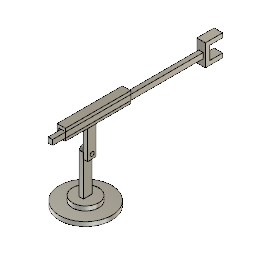
Modelling and Simulation of a Polar Robot (RRP) (Autodesk Fusion 360 design; units mm, degrees)
Autodesk Fusion 360 part; units mm, degrees
sketch "Sketch1" plane through (0, 0, 0) normal (0, 0, 1) x (1, 0, 0)
  circle A0 centre (0, 0) radius 60
  dimension "d1" = 120
  constraint coincident A0.centre origin
  measures "d1" diameter of A0
extrude "Extrude1" add sketch "Sketch1" along normal blind 10 makes body 1 in component "Component"
sketch "Sketch2" plane through (0, 0, 10) normal (0, 0, 1) x (-1, 0, 0)
  circle A0 centre (0, 0) radius 60
  circle A1 centre (0, 0) radius 30
  dimension "d4" = 60
  constraint coincident A0.centre A1.centre
  measures "d4" diameter of A1
extrude "Extrude1'" add sketch "Sketch2" along normal blind 10 separate body contours A1 makes body 2 in component "Component'"
sketch "Sketch3" plane through (0, 0, 20) normal (0, 0, 1) x (-1, 0, 0)
  circle A0 centre (0, 0) radius 30
  line L0 (-5, 10) -> (5, 10)
  line L1 (5, 10) -> (5, -10)
  line L2 (5, -10) -> (-5, -10)
  line L3 (-5, -10) -> (-5, 10)
  line L4 (-5, 10) -> (5, -10) construction
  line L5 (5, 10) -> (-5, -10) construction
  dimension "d7" = 20
  dimension "d8" = 10
  dimension "d9" = 10
  dimension "d10" = 20
  constraint horizontal L0
  constraint perpendicular L0 L1
  constraint parallel L0 L2
  constraint parallel L1 L3
  constraint coincident L4 A0.centre
  constraint coincident L5 A0.centre
  constraint coincident A0.centre origin
  measures "d7" distance of L0.end L1.end
  measures "d8" distance of L1.end L2.end
  measures "d9" distance of L1.end L2.end
  measures "d10" distance of L0.end L1.end
extrude "Extrude2" add sketch "Sketch3" along normal blind 100 contours L0 L1 L2 L3 bodies 2 in component "Component'"
sketch "Sketch4" plane through (-5, 0, 0) normal (-1, 0, 0) x (0, -1, 0)
  line L0 (-10, 20) -> (10, 20)
  line L1 (10, 20) -> (10, 120)
  line L2 (10, 120) -> (-10, 120)
  line L3 (-10, 120) -> (-10, 20)
  arc A0 (10, 106.2063) -> (-10, 105.8869) centre (-0.0542, 109.439) ccw
  line L4 (-10, 105.8869) -> (-10, 120)
  line L5 (10, 120) -> (10, 106.2063)
  constraint coincident L1 A0.start
  constraint coincident L3 A0.end
  constraint coincident L2.end L3.start
  constraint coincident L1.end L2.start
extrude "Extrude3" cut sketch "Sketch4" against normal blind 70 contours L2 L3 A0 L4 | L1 L2 A0 L5 bodies 2 in component "Component'"
sketch "Sketch5" plane through (5, 0, 0) normal (1, 0, 0) x (0, 1, 0)
  arc A0 (10, 112.9912) -> (0.1084, 120) centre (0.0542, 109.439) ccw
  line L0 (0.1084, 120) -> (0, 120)
  arc A1 (0, 120) -> (-10, 112.6717) centre (0.0542, 109.439) ccw
  line L1 (-10, 112.6717) -> (-10, 20)
  line L2 (-10, 20) -> (10, 20)
  line L3 (10, 20) -> (10, 112.9912)
  circle A2 centre (0.0542, 109.439) radius 4.5
  dimension "d15" = 9
  constraint concentric A0 A2
  measures "d15" diameter of A2
extrude "Extrude4" add sketch "Sketch5" along normal blind 10 contours A2 bodies 2 in component "Component'"
sketch "Sketch6" plane through (15, 0, 0) normal (1, 0, 0) x (0, 1, 0)
  circle A0 centre (0.0542, 109.439) radius 4.5
  line L0 (-10, 120) -> (60, 120)
  line L1 (60, 120) -> (60, 100)
  line L2 (60, 100) -> (-10, 100)
  line L3 (-10, 100) -> (-10, 120)
  constraint horizontal L0
  constraint vertical L1
  constraint horizontal L2
  constraint vertical L3
extrude "Extrude1''" add sketch "Sketch6" against normal blind 10 separate body makes body 3 in component "Component''"
sketch "Sketch7" plane through (0, 9.4932, 0) normal (0, 1, 0) x (-1, 0, 0)
  line L0 (-15, 169.3849) -> (-15, 99.3849)
  line L1 (-15, 99.3849) -> (-5, 99.3849)
  line L2 (-5, 99.3849) -> (-5, 169.3849)
  line L3 (-5, 169.3849) -> (-15, 169.3849)
  line L4 (-19.341, 169.3448) -> (0.1035, 169.3448)
  line L5 (0.1035, 169.3448) -> (0.1035, 195.3844)
  line L6 (0.1035, 195.3844) -> (-19.341, 195.3844)
  line L7 (-19.341, 195.3844) -> (-19.341, 169.3448)
  line L8 (-19.341, 169.3448) -> (0.1035, 195.3844) construction
  line L9 (0.1035, 169.3448) -> (-19.341, 195.3844) construction
  point P0 (-9.6187, 182.3646)
  constraint horizontal L4
  constraint perpendicular L4 L5
  constraint parallel L4 L6
  constraint parallel L5 L7
  constraint coincident L8 P0
  constraint coincident L9 P0
extrude "Extrude2'" add sketch "Sketch7" along normal mid plane 150 contours L0 L2 L3 L4 L5 L6 L7 sketch seen with x (1, 0, 0) y (0, 0, -1) z (0, 1, 0) at (0, -109.3849, 109.4932) bodies 3 in component "Component''"
sketch "Sketch8" plane through (0, 84.4932, 0) normal (0, 1, 0) x (-1, 0, 0)
  line L0 (-5, 169.3448) -> (0.1035, 169.3448)
  line L1 (0.1035, 169.3448) -> (0.1035, 195.3844)
  line L2 (0.1035, 195.3844) -> (-19.341, 195.3844)
  line L3 (-19.341, 195.3844) -> (-19.341, 169.3448)
  line L4 (-19.341, 169.3448) -> (-15, 169.3448)
  line L5 (-15, 169.3448) -> (-15, 169.3849)
  line L6 (-15, 169.3849) -> (-5, 169.3849)
  line L7 (-5, 169.3849) -> (-5, 169.3448)
  line L8 (-4.1596, 176.2347) -> (-14.668, 176.2347)
  line L9 (-14.668, 176.2347) -> (-14.668, 188.4945)
  line L10 (-14.668, 188.4945) -> (-4.1596, 188.4945)
  line L11 (-4.1596, 188.4945) -> (-4.1596, 176.2347)
  line L12 (-4.1596, 176.2347) -> (-14.668, 188.4945) construction
  line L13 (-14.668, 176.2347) -> (-4.1596, 188.4945) construction
  point P0 (-9.4138, 182.3646)
  constraint horizontal L8
  constraint perpendicular L8 L9
  constraint parallel L8 L10
  constraint parallel L9 L11
  constraint coincident L12 P0
  constraint coincident L13 P0
extrude "Extrude3'" cut sketch "Sketch8" against normal blind 330 contours L8 L9 L10 L11 sketch seen with x (1, 0, 0) y (0, 0, -1) z (0, 1, 0) at (0, -109.3849, 109.4932) bodies 3 in component "Component''"
sketch "Sketch9" plane through (0, 84.4932, 0) normal (0, 1, 0) x (-1, 0, 0)
  line L0 (-14.668, 176.2347) -> (-14.668, 188.4945)
  line L1 (-14.668, 188.4945) -> (-4.1596, 188.4945)
  line L2 (-4.1596, 188.4945) -> (-4.1596, 176.2347)
  line L3 (-4.1596, 176.2347) -> (-14.668, 176.2347)
  line L4 (-5, 169.3448) -> (0.1035, 169.3448)
  line L5 (0.1035, 169.3448) -> (0.1035, 195.3844)
  line L6 (0.1035, 195.3844) -> (-19.341, 195.3844)
  line L7 (-19.341, 195.3844) -> (-19.341, 169.3448)
  line L8 (-19.341, 169.3448) -> (-15, 169.3448)
  line L9 (-15, 169.3448) -> (-15, 169.3849)
  line L10 (-15, 169.3849) -> (-5, 169.3849)
  line L11 (-5, 169.3849) -> (-5, 169.3448)
  line L12 (-14.668, 188.4945) -> (-4.1596, 188.4945)
  line L13 (-4.1596, 188.4945) -> (-4.1596, 176.2347)
  line L14 (-4.1596, 176.2347) -> (-14.668, 176.2347)
  line L15 (-14.668, 176.2347) -> (-14.668, 188.4945)
  constraint horizontal L12
  constraint vertical L13
  constraint horizontal L14
  constraint vertical L15
  constraint coincident L2.end L3.start
  constraint coincident L0.end L1.start
extrude "Extrude1'''" add sketch "Sketch9" against normal blind 360 separate body contours L0 L1 L2 L3 L12 L13 L14 L15 makes body 4 in component "Component'''"
ref_plane "WorkPlane1" through (14.668, 84.4932, 182.3646) normal (1, 0, 0) x (0, 0, 1)
sketch "Sketch10" plane through (14.668, 0, 0) normal (1, 0, 0) x (0, 1, 0)
  line L0 (250, 210) -> (290, 210)
  line L1 (290, 160) -> (250, 160)
  line L2 (250, 160) -> (250, 210)
  line L3 (260, 200) -> (290, 200)
  line L4 (290, 170) -> (260, 170)
  line L5 (260, 170) -> (260, 200)
  line L6 (290, 210) -> (290, 200)
  line L7 (290, 170) -> (290, 160)
  constraint horizontal L0
  constraint vertical L6
  constraint horizontal L1
  constraint vertical L2
  constraint horizontal L3
  constraint horizontal L4
  constraint vertical L5
  constraint collinear L6 L7
extrude "Extrude2''" add sketch "Sketch10" along normal mid plane 20 sketch seen with x (1, 0, 0) y (0, 1, 0) z (0, 0, 1) at (-5.2542, -180, 0) bodies 4 in component "Component'''"
component "Component" placed x (1, 0, 0) y (0, 1, 0) z (0, 0, 1) at (0, 0, 0)
component "Component'" placed x (1, 0, 0) y (0, 1, 0) z (0, 0, 1) at (0, 0, 0)
component "Component''" placed x (1, 0, 0) y (0, 0, 1) z (0, -1, 0) at (0, 109.4932, 109.3849)
component "Component'''" placed x (1, 0, 0) y (0, 1, 0) z (0, 0, 1) at (5.2542, 180, 0)
